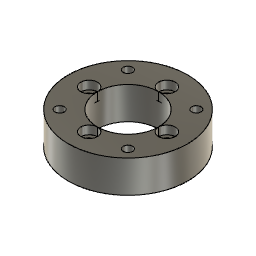
Z_Axis_Nema17_Adaptor (Autodesk Fusion 360 design; units mm, degrees)
Autodesk Fusion 360 part; units mm, degrees
sketch "Sketch1" plane through (0, 0, 0) normal (0, 0, 1) x (1, 0, 0)
  circle A0 centre (0.0122, 0.0049) radius 21.59
  circle A1 centre (-12.3626, -12.3699) radius 1.666
  circle A2 centre (12.387, 12.3797) radius 1.666
  circle A3 centre (12.387, -12.3699) radius 1.666
  circle A4 centre (-12.3626, 12.3797) radius 1.666
  circle A5 centre (0.0122, 0.0049) radius 17.9705 construction
  circle A6 centre (0.0122, 0.0049) radius 11.049
  circle A7 centre (14.0713, 0.0049) radius 1.6637
  circle A8 centre (0.0122, 14.0641) radius 1.6637
  circle A9 centre (-14.047, 0.0049) radius 1.6637
  circle A10 centre (0.0122, -14.0542) radius 1.6637
  circle A11 centre (14.0713, 0.0049) radius 3.0102
  circle A12 centre (0.0122, 14.0641) radius 3.0102
  circle A13 centre (-14.047, 0.0049) radius 3.0102
  circle A14 centre (0.0122, -14.0542) radius 3.0102
  dimension "d4" = 3.3274
  dimension "d6" = 360
  constraint concentric A7 A11
  constraint tangent A6 A11
  constraint concentric A8 A12
  constraint tangent A6 A12
  constraint concentric A9 A13
  constraint tangent A6 A13
  constraint concentric A10 A14
  constraint tangent A6 A14
  measures "d4" diameter of A7
extrude "Extrude1" add sketch "Sketch1" against normal blind 11.684 contours A0 | A14 | A13 | A12 | A11
extrude "Extrude2" cut sketch "Sketch1" against normal blind 3.048 contours A14 | A13 | A12 | A11
